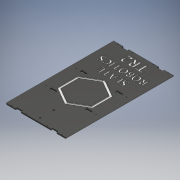
# Autodesk Inventor part: BA11
Saved by Autodesk Inventor 2017 (Build 210142000, 142)
## iProperties
Created: 2019-05-29
Part Number: BA11
Material: Wood (Cherry)
Document SubType Name: Modeling
Designer: Dell
Density: 0.63 g/cm^3
Appearance: Smooth - Black
Mass: 641.872 g
Surface Area: 3346.2 cm^2
Volume: 1018.84 cm^3
Author: Dell
Autodesk Inventor part; units mm, degrees
ref_plane "YZ Plane" through (0, 0, 0) normal (1, 0, 0) x (0, 1, 0)
ref_plane "XZ Plane" through (0, 0, 0) normal (0, 1, 0) x (-1, 0, 0)
ref_plane "XY Plane" through (0, 0, 0) normal (0, 0, 1) x (1, 0, 0)
sketch "Sketch1" plane through (0, 0, 0) normal (0, 0, 1) x (1, 0, 0)
  line L0 (0, 0) -> (303.5592, 0)
  line L1 (303.5592, 0) -> (303.5592, 539.75)
  line L2 (303.5592, 539.75) -> (0, 539.75)
  line L3 (0, 539.75) -> (0, 0)
  dimension "d0" = 539.75
  dimension "d1" = 303.5592
  constraints: 8 end point, 2 parallel, 1 horizontal, 1 perpendicular
  measures "d0" distance of L1.end L0.end
  measures "d1" distance of L1.end L2.end
extrude "Extrusion1" add sketch "Sketch1" along normal blind 6.35
sketch "Sketch2" plane through (0, 539.75, 0) normal (0, 1, 0) x (1, 0, 0)
  line L0 (0, -6.35) -> (303.5592, -6.35) projected
  line L1 (0, -6.35) -> (3.6662, 0)
  line L2 (0, 0) -> (303.5592, 0) projected
  line L3 (0, 0) -> (3.6662, 0)
  line L4 (0, 0) -> (0, -6.35)
  line L5 (303.5592, -6.35) -> (299.8931, 0)
  line L6 (303.5592, 0) -> (299.8931, 0)
  line L7 (303.5592, 0) -> (303.5592, -6.35) projected
  line L8 (303.5592, 0) -> (303.5592, -6.35)
  dimension "d4" = 30
  dimension "d5" = 30
  constraints: 12 end point, 2 collinear, 2 point on line, 1 perpendicular, 1 vertical
  measures "d4" angle of L4 L1
  measures "d5" angle of L5 L7
extrude "Extrusion2" cut sketch "Sketch2" against normal through all contours L4 L2 L1 | L5 L2 L7
sketch "Sketch3" plane through (0, 0, 6.35) normal (0, 0, 1) x (1, 0, 0)
  line L0 (50.1796, 532.13) -> (75.5796, 532.13)
  line L1 (75.5796, 532.13) -> (75.5796, 539.75)
  line L2 (75.5796, 539.75) -> (50.1796, 539.75)
  line L3 (50.1796, 539.75) -> (50.1796, 532.13)
  line L4 (303.5592, 539.75) -> (0, 539.75) projected
  line L5 (227.9796, 539.75) -> (253.3796, 539.75)
  line L6 (253.3796, 539.75) -> (253.3796, 532.13)
  line L7 (253.3796, 532.13) -> (227.9796, 532.13)
  line L8 (227.9796, 532.13) -> (227.9796, 539.75)
  line L9 (75.5796, 532.13) -> (227.9796, 532.13) construction
  line L10 (0, 0) -> (303.5592, 0) projected
  line L11 (50.1796, 0) -> (75.5796, 0)
  line L12 (75.5796, 0) -> (75.5796, 7.62)
  line L13 (75.5796, 7.62) -> (50.1796, 7.62)
  line L14 (50.1796, 7.62) -> (50.1796, 0)
  line L15 (253.3796, 0) -> (227.9796, 0)
  line L16 (227.9796, 0) -> (227.9796, 7.62)
  line L17 (227.9796, 7.62) -> (253.3796, 7.62)
  line L18 (253.3796, 7.62) -> (253.3796, 0)
  point P0 (151.7796, 532.13)
  point P1 (151.7796, 539.75)
  dimension "d8" = 7.62
  dimension "d9" = 25.4
  dimension "d10" = 25.4
  dimension "d11" = 152.4
  dimension "d14" = 7.62
  constraints: 34 end point, 8 parallel, 5 point on line, 5 vertical alignment, 4 horizontal, 4 perpendicular, 2 midpoint, 1 collinear, 1 horizontal alignment
  measures "d8" distance of L2.end L0.start
  measures "d9" distance of L0.start L0.end
  measures "d10" distance of L6.end L7.end
  measures "d11" distance of L0.end L7.end
  measures "d14" distance of L13.end L11.start
extrude "Extrusion3" cut sketch "Sketch3" against normal through all
sketch "Sketch4" plane through (0, 0, 6.35) normal (0, 0, 1) x (1, 0, 0)
  line L0 (50.1796, 330.2) -> (75.5796, 330.2)
  line L1 (75.5796, 330.2) -> (75.5796, 323.85)
  line L2 (75.5796, 323.85) -> (50.1796, 323.85)
  line L3 (50.1796, 323.85) -> (50.1796, 330.2)
  line L4 (227.9796, 330.2) -> (253.3796, 330.2)
  line L5 (253.3796, 330.2) -> (253.3796, 323.85)
  line L6 (253.3796, 323.85) -> (227.9796, 323.85)
  line L7 (227.9796, 323.85) -> (227.9796, 330.2)
  line L8 (75.5796, 532.13) -> (50.1796, 532.13) projected
  line L9 (253.3796, 532.13) -> (227.9796, 532.13) projected
  line L10 (227.9796, 539.75) -> (75.5796, 539.75) projected
  point P0 (0, 0)
  point P1 (62.8796, 330.2)
  point P2 (62.8796, 532.13)
  point P3 (240.6796, 330.2)
  point P4 (240.6796, 532.13)
  dimension "d15" = 25.4
  dimension "d16" = 6.35
  dimension "d17" = 25.4
  dimension "d18" = 6.35
  dimension "d19" = 209.55
  constraints: 16 end point, 4 midpoint, 4 parallel, 2 horizontal, 2 perpendicular, 2 vertical alignment, 1 horizontal alignment
  measures "d15" distance of L1.end L2.end
  measures "d16" distance of L0.end L1.end
  measures "d17" distance of L5.end L6.end
  measures "d18" distance of L4.end L5.end
  measures "d19" distance between parallel lines of L10 L0
extrude "Extrusion4" cut sketch "Sketch4" against normal through all
sketch "Sketch5" plane through (0, 0, 6.35) normal (0, 0, 1) x (1, 0, 0)
  line L0 (50.1796, 177.8) -> (75.5796, 177.8)
  line L1 (75.5796, 177.8) -> (75.5796, 171.45)
  line L2 (75.5796, 171.45) -> (50.1796, 171.45)
  line L3 (50.1796, 171.45) -> (50.1796, 177.8)
  line L4 (227.9796, 177.8) -> (253.3796, 177.8)
  line L5 (253.3796, 177.8) -> (253.3796, 171.45)
  line L6 (253.3796, 171.45) -> (227.9796, 171.45)
  line L7 (227.9796, 171.45) -> (227.9796, 177.8)
  line L8 (50.1796, 7.62) -> (75.5796, 7.62) projected
  line L9 (227.9796, 7.62) -> (253.3796, 7.62) projected
  line L10 (0, 0) -> (50.1796, 0) projected
  point P0 (62.8796, 171.45)
  point P1 (62.8796, 7.62)
  point P2 (240.6796, 7.62)
  point P3 (240.6796, 171.45)
  dimension "d22" = 25.4
  dimension "d23" = 6.35
  dimension "d24" = 25.4
  dimension "d25" = 6.35
  dimension "d27" = 177.8
  constraints: 16 end point, 4 midpoint, 4 parallel, 2 horizontal, 2 perpendicular, 2 vertical alignment, 1 horizontal alignment
  measures "d22" distance of L1.end L2.end
  measures "d23" distance of L0.end L1.end
  measures "d24" distance of L5.end L6.end
  measures "d25" distance of L4.end L5.end
  measures "d27" distance between parallel lines of L10 L0
extrude "Extrusion5" cut sketch "Sketch5" against normal through all
sketch "Sketch6" plane through (0, 0, 6.35) normal (0, 0, 1) x (1, 0, 0)
  line L0 (301.7796, 364.75) -> (1.7796, 364.75) construction
  line L1 (1.7796, 364.75) -> (1.7796, 514.75) construction
  line L2 (301.7796, 514.75) -> (301.7796, 364.75) construction
  line L3 (1.7796, 514.75) -> (301.7796, 514.75) construction
  line L4 (151.7796, 364.75) -> (151.7796, 439.75) construction
  line L5 (151.7796, 439.75) -> (1.7796, 439.75) construction
  line L6 (227.9796, 539.75) -> (75.5796, 539.75) projected
  line L7 (151.7796, 143.9637) -> (64.2796, 194.4819)
  line L8 (64.2796, 194.4819) -> (64.2796, 295.5181)
  line L9 (64.2796, 295.5181) -> (151.7796, 346.0363)
  line L10 (151.7796, 346.0363) -> (239.2796, 295.5181)
  line L11 (239.2796, 295.5181) -> (239.2796, 194.4819)
  line L12 (239.2796, 194.4819) -> (151.7796, 143.9637)
  line L13 (151.7796, 155.7416) -> (74.4796, 200.3708)
  line L14 (74.4796, 200.3708) -> (74.4796, 289.6292)
  line L15 (74.4796, 289.6292) -> (151.7796, 334.2584)
  line L16 (151.7796, 334.2584) -> (229.0796, 289.6292)
  line L17 (229.0796, 289.6292) -> (229.0796, 200.3708)
  line L18 (229.0796, 200.3708) -> (151.7796, 155.7416)
  line L19 (75.5796, 0) -> (227.9796, 0) projected
  line L20 (221.0068, 398.0391) -> (221.0068, 392.4691)
  spline S0 degree 2 poles (221.0068, 392.4691) (217.2023, 394.0605) (213.4476, 394.6822) (211.881, 394.6822) knots 0 0 0 1 2 2 2
  spline S1 degree 2 poles (211.881, 394.6822) (209.0463, 394.6822) (206.2364, 392.1458) (206.2364, 390.3555) knots 0 0 0 1 2 2 2
  spline S2 degree 2 poles (206.2364, 390.3555) (206.2364, 388.9878) (207.0072, 387.8937) knots 0 0 0 1 1 1
  spline S3 degree 2 poles (207.0072, 387.8937) (207.8029, 386.8245) (210.8615, 385.1087) knots 0 0 0 1 1 1
  line L21 (210.8615, 385.1087) -> (213.0497, 383.8903)
  spline S4 degree 2 poles (213.0497, 383.8903) (217.7494, 381.2793) (219.3906, 379.0663) knots 0 0 0 1 1 1
  spline S5 degree 2 poles (219.3906, 379.0663) (221.0814, 376.8532) (221.0814, 373.9438) knots 0 0 0 1 1 1
  spline S6 degree 2 poles (221.0814, 373.9438) (221.0814, 370.2637) (215.4617, 365.0418) (210.215, 365.0418) knots 0 0 0 1 2 2 2
  spline S7 degree 2 poles (210.215, 365.0418) (206.2861, 365.0418) (201.3626, 366.1607) knots 0 0 0 1 1 1
  line L22 (201.3626, 366.1607) -> (201.3626, 371.3578)
  spline S8 degree 2 poles (201.3626, 371.3578) (206.4104, 369.4928) (209.3695, 369.4928) knots 0 0 0 1 1 1
  spline S9 degree 2 poles (209.3695, 369.4928) (211.8313, 369.4928) (214.3925, 371.6313) (214.3925, 373.1233) knots 0 0 0 1 2 2 2
  spline S10 degree 2 poles (214.3925, 373.1233) (214.3925, 374.2671) (213.5968, 375.2369) knots 0 0 0 1 1 1
  spline S11 degree 2 poles (213.5968, 375.2369) (212.8508, 376.2315) (209.7922, 377.9473) knots 0 0 0 1 1 1
  line L23 (209.7922, 377.9473) -> (207.4548, 379.2403)
  spline S12 degree 2 poles (207.4548, 379.2403) (202.0589, 382.2491) (200.5918, 384.4622) knots 0 0 0 1 1 1
  spline S13 degree 2 poles (200.5918, 384.4622) (199.1247, 386.7002) (199.1247, 389.4852) knots 0 0 0 1 1 1
  spline S14 degree 2 poles (199.1247, 389.4852) (199.1247, 393.4886) (205.2169, 399.1332) (211.8561, 399.1332) knots 0 0 0 1 2 2 2
  spline S15 degree 2 poles (211.8561, 399.1332) (215.785, 399.1332) (221.0068, 398.0391) knots 0 0 0 1 1 1
  line L24 (193.5049, 398.3375) -> (193.5049, 365.8375)
  line L25 (193.5049, 365.8375) -> (186.7414, 365.8375)
  line L26 (186.7414, 365.8375) -> (186.7414, 393.7373)
  line L27 (186.7414, 393.7373) -> (172.2444, 393.7373)
  line L28 (172.2444, 393.7373) -> (172.2444, 398.3375)
  line L29 (172.2444, 398.3375) -> (193.5049, 398.3375)
  line L30 (170.9265, 398.3375) -> (158.3194, 365.8375)
  line L31 (158.3194, 365.8375) -> (151.531, 365.8375)
  line L32 (151.531, 365.8375) -> (138.8741, 398.3375)
  line L33 (138.8741, 398.3375) -> (145.8117, 398.3375)
  line L34 (145.8117, 398.3375) -> (149.1935, 389.6592)
  line L35 (149.1935, 389.6592) -> (162.6212, 389.6592)
  line L36 (162.6212, 389.6592) -> (166.003, 398.3375)
  line L37 (166.003, 398.3375) -> (170.9265, 398.3375)
  line L38 (160.9552, 385.3325) -> (150.8844, 385.3325)
  line L39 (150.8844, 385.3325) -> (155.9074, 372.3773)
  line L40 (155.9074, 372.3773) -> (160.9552, 385.3325)
  line L41 (126.1924, 398.3375) -> (126.1924, 370.3134)
  line L42 (126.1924, 370.3134) -> (137.8297, 370.3134)
  line L43 (137.8297, 370.3134) -> (137.8297, 365.8375)
  line L44 (137.8297, 365.8375) -> (107.7915, 365.8375)
  line L45 (107.7915, 365.8375) -> (107.7915, 370.3134)
  line L46 (107.7915, 370.3134) -> (119.4288, 370.3134)
  line L47 (119.4288, 370.3134) -> (119.4288, 398.3375)
  line L48 (119.4288, 398.3375) -> (126.1924, 398.3375)
  line L49 (103.2658, 398.3375) -> (103.2658, 365.8375)
  line L50 (103.2658, 365.8375) -> (82.4529, 365.8375)
  line L51 (82.4529, 365.8375) -> (82.4529, 370.3134)
  line L52 (82.4529, 370.3134) -> (96.5023, 370.3134)
  line L53 (96.5023, 370.3134) -> (96.5023, 379.3646)
  line L54 (96.5023, 379.3646) -> (84.8898, 379.3646)
  line L55 (84.8898, 379.3646) -> (84.8898, 383.8405)
  line L56 (84.8898, 383.8405) -> (96.5023, 383.8405)
  line L57 (96.5023, 383.8405) -> (96.5023, 393.7373)
  line L58 (96.5023, 393.7373) -> (81.4085, 393.7373)
  line L59 (81.4085, 393.7373) -> (81.4085, 398.3375)
  line L60 (81.4085, 398.3375) -> (103.2658, 398.3375)
  line L61 (266.201, 450.2809) -> (266.201, 417.7809)
  line L62 (266.201, 417.7809) -> (254.0415, 417.7809)
  spline S16 degree 2 poles (254.0415, 417.7809) (250.3116, 417.7809) (246.4076, 419.6459) (244.1448, 423.4504) (244.1448, 425.8376) knots 0 0 0 1 2 3 3 3
  spline S17 degree 2 poles (244.1448, 425.8376) (244.1448, 428.6972) (247.4271, 433.7699) (250.4359, 435.1126) knots 0 0 0 1 2 2 2
  line L63 (250.4359, 435.1126) -> (239.8181, 450.2809)
  line L64 (239.8181, 450.2809) -> (248.0487, 450.2809)
  line L65 (248.0487, 450.2809) -> (256.1302, 437.0024)
  line L66 (256.1302, 437.0024) -> (259.8353, 437.0024)
  line L67 (259.8353, 437.0024) -> (259.8353, 450.2809)
  line L68 (259.8353, 450.2809) -> (266.201, 450.2809)
  line L69 (259.8353, 432.5514) -> (258.2936, 432.5514)
  spline S18 degree 2 poles (258.2936, 432.5514) (254.1161, 432.5514) (250.9083, 428.8961) (250.9083, 426.5835) knots 0 0 0 1 2 2 2
  spline S19 degree 2 poles (250.9083, 426.5835) (250.9083, 424.5943) (253.4944, 422.232) (257.473, 422.232) knots 0 0 0 1 2 2 2
  line L70 (257.473, 422.232) -> (259.8353, 422.232)
  line L71 (259.8353, 422.232) -> (259.8353, 432.5514)
  spline S20 degree 2 poles (220.7209, 451.0767) (225.7936, 451.0767) (233.3031, 446.8743) (237.2071, 439.0166) (237.2071, 434.0185) knots 0 0 0 1 2 3 3 3
  spline S21 degree 2 poles (237.2071, 434.0185) (237.2071, 429.0702) (233.3031, 421.1627) (225.7438, 416.9852) (220.7209, 416.9852) knots 0 0 0 1 2 3 3 3
  spline S22 degree 2 poles (220.7209, 416.9852) (215.7228, 416.9852) (208.1635, 421.1627) (204.2595, 429.0702) (204.2595, 434.0185) knots 0 0 0 1 2 3 3 3
  spline S23 degree 2 poles (204.2595, 434.0185) (204.2595, 439.0166) (208.1635, 446.8743) (215.6482, 451.0767) (220.7209, 451.0767) knots 0 0 0 1 2 3 3 3
  spline S24 degree 2 poles (220.7209, 446.6256) (216.0212, 446.6256) (211.4458, 438.9669) (211.4458, 434.0185) knots 0 0 0 1 2 2 2
  spline S25 degree 2 poles (211.4458, 434.0185) (211.4458, 429.0453) (216.0461, 421.4363) (220.7209, 421.4363) knots 0 0 0 1 2 2 2
  spline S26 degree 2 poles (220.7209, 421.4363) (225.4206, 421.4363) (230.0208, 429.0453) (230.0208, 434.0185) knots 0 0 0 1 2 2 2
  spline S27 degree 2 poles (230.0208, 434.0185) (230.0208, 438.9669) (225.4454, 446.6256) (220.7209, 446.6256) knots 0 0 0 1 2 2 2
  line L72 (198.1922, 450.2809) -> (198.1922, 417.7809)
  line L73 (198.1922, 417.7809) -> (187.2262, 417.7809)
  spline S28 degree 2 poles (187.2262, 417.7809) (183.2477, 417.7809) (179.4432, 419.5713) (177.2798, 423.0526) (177.2798, 425.017) knots 0 0 0 1 2 3 3 3
  spline S29 degree 2 poles (177.2798, 425.017) (177.2798, 427.4539) (180.6616, 431.9298) (185.038, 433.2974) knots 0 0 0 1 2 2 2
  spline S30 degree 2 poles (185.038, 433.2974) (181.5568, 434.1677) (177.8766, 436.7041) (175.9619, 440.235) (175.9619, 442.2492) knots 0 0 0 1 2 3 3 3
  spline S31 degree 2 poles (175.9619, 442.2492) (175.9619, 444.4374) (178.1998, 448.2419) (182.1287, 450.2809) (186.2067, 450.2809) knots 0 0 0 1 2 3 3 3
  line L74 (186.2067, 450.2809) -> (198.1922, 450.2809)
  line L75 (191.7021, 445.6807) -> (190.4091, 445.6807)
  spline S32 degree 2 poles (190.4091, 445.6807) (186.8781, 445.6807) (184.3169, 444.7607) (183.0239, 442.6968) (183.0239, 441.4286) knots 0 0 0 1 2 3 3 3
  spline S33 degree 2 poles (183.0239, 441.4286) (183.0239, 439.0166) (187.276, 435.6597) (190.5334, 435.6597) knots 0 0 0 1 2 2 2
  line L76 (190.5334, 435.6597) -> (191.7021, 435.6597)
  line L77 (191.7021, 435.6597) -> (191.7021, 445.6807)
  line L78 (191.7021, 431.3081) -> (190.2599, 431.3081)
  spline S34 degree 2 poles (190.2599, 431.3081) (187.1765, 431.3081) (184.1428, 428.2496) (184.1428, 426.0614) knots 0 0 0 1 2 2 2
  spline S35 degree 2 poles (184.1428, 426.0614) (184.1428, 424.8927) (185.038, 423.1769) (187.3008, 422.232) (190.4837, 422.232) knots 0 0 0 1 2 3 3 3
  line L79 (190.4837, 422.232) -> (191.7021, 422.232)
  line L80 (191.7021, 422.232) -> (191.7021, 431.3081)
  spline S36 degree 2 poles (155.3976, 451.0767) (160.4703, 451.0767) (167.9799, 446.8743) (171.8839, 439.0166) (171.8839, 434.0185) knots 0 0 0 1 2 3 3 3
  spline S37 degree 2 poles (171.8839, 434.0185) (171.8839, 429.0702) (167.9799, 421.1627) (160.4206, 416.9852) (155.3976, 416.9852) knots 0 0 0 1 2 3 3 3
  spline S38 degree 2 poles (155.3976, 416.9852) (150.3995, 416.9852) (142.8402, 421.1627) (138.9363, 429.0702) (138.9363, 434.0185) knots 0 0 0 1 2 3 3 3
  spline S39 degree 2 poles (138.9363, 434.0185) (138.9363, 439.0166) (142.8402, 446.8743) (150.3249, 451.0767) (155.3976, 451.0767) knots 0 0 0 1 2 3 3 3
  spline S40 degree 2 poles (155.3976, 446.6256) (150.6979, 446.6256) (146.1226, 438.9669) (146.1226, 434.0185) knots 0 0 0 1 2 2 2
  spline S41 degree 2 poles (146.1226, 434.0185) (146.1226, 429.0453) (150.7228, 421.4363) (155.3976, 421.4363) knots 0 0 0 1 2 2 2
  spline S42 degree 2 poles (155.3976, 421.4363) (160.0973, 421.4363) (164.6976, 429.0453) (164.6976, 434.0185) knots 0 0 0 1 2 2 2
  spline S43 degree 2 poles (164.6976, 434.0185) (164.6976, 438.9669) (160.1222, 446.6256) (155.3976, 446.6256) knots 0 0 0 1 2 2 2
  line L81 (124.7875, 450.2809) -> (124.7875, 422.2568)
  line L82 (124.7875, 422.2568) -> (136.4248, 422.2568)
  line L83 (136.4248, 422.2568) -> (136.4248, 417.7809)
  line L84 (136.4248, 417.7809) -> (106.3865, 417.7809)
  line L85 (106.3865, 417.7809) -> (106.3865, 422.2568)
  line L86 (106.3865, 422.2568) -> (118.0239, 422.2568)
  line L87 (118.0239, 422.2568) -> (118.0239, 450.2809)
  line L88 (118.0239, 450.2809) -> (124.7875, 450.2809)
  line L89 (101.8609, 450.2809) -> (101.8609, 417.7809)
  line L90 (101.8609, 417.7809) -> (95.0973, 417.7809)
  line L91 (95.0973, 417.7809) -> (95.0973, 450.2809)
  line L92 (95.0973, 450.2809) -> (101.8609, 450.2809)
  spline S44 degree 2 poles (60.807, 448.9879) (62.9454, 449.9328) (66.1034, 450.6291) (70.1069, 451.0767) (72.0713, 451.0767) knots 0 0 0 1 2 3 3 3
  spline S45 degree 2 poles (72.0713, 451.0767) (80.6004, 451.0767) (88.9803, 441.4783) (88.9803, 434.0185) knots 0 0 0 1 2 2 2
  spline S46 degree 2 poles (88.9803, 434.0185) (88.9803, 426.5587) (80.6253, 416.9852) (71.6486, 416.9852) knots 0 0 0 1 2 2 2
  spline S47 degree 2 poles (71.6486, 416.9852) (66.3521, 416.9852) (61.1054, 418.2285) knots 0 0 0 1 1 1
  line L93 (61.1054, 418.2285) -> (61.1054, 423.525)
  spline S48 degree 2 poles (61.1054, 423.525) (63.6417, 422.6547) (66.8494, 421.8341) (69.709, 421.4363) (71.1513, 421.4363) knots 0 0 0 1 2 3 3 3
  spline S49 degree 2 poles (71.1513, 421.4363) (76.7461, 421.4363) (81.794, 428.6226) (81.794, 433.9439) knots 0 0 0 1 2 2 2
  spline S50 degree 2 poles (81.794, 433.9439) (81.794, 439.5139) (76.0748, 446.4018) (70.4053, 446.4018) knots 0 0 0 1 2 2 2
  spline S51 degree 2 poles (70.4053, 446.4018) (65.6807, 446.4018) (60.807, 444.0147) knots 0 0 0 1 1 1
  line L94 (60.807, 444.0147) -> (60.807, 448.9879)
  line L95 (56.7538, 449.9826) -> (56.7538, 444.4125)
  spline S52 degree 2 poles (56.7538, 444.4125) (52.9493, 446.004) (49.1945, 446.6256) (47.6279, 446.6256) knots 0 0 0 1 2 2 2
  spline S53 degree 2 poles (47.6279, 446.6256) (44.7932, 446.6256) (41.9833, 444.0893) (41.9833, 442.2989) knots 0 0 0 1 2 2 2
  spline S54 degree 2 poles (41.9833, 442.2989) (41.9833, 440.9313) (42.7542, 439.8372) knots 0 0 0 1 1 1
  spline S55 degree 2 poles (42.7542, 439.8372) (43.5499, 438.7679) (46.6084, 437.0522) knots 0 0 0 1 1 1
  line L96 (46.6084, 437.0522) -> (48.7966, 435.8337)
  spline S56 degree 2 poles (48.7966, 435.8337) (53.4963, 433.2228) (55.1375, 431.0097) knots 0 0 0 1 1 1
  spline S57 degree 2 poles (55.1375, 431.0097) (56.8284, 428.7966) (56.8284, 425.8873) knots 0 0 0 1 1 1
  spline S58 degree 2 poles (56.8284, 425.8873) (56.8284, 422.2071) (51.2086, 416.9852) (45.9619, 416.9852) knots 0 0 0 1 2 2 2
  spline S59 degree 2 poles (45.9619, 416.9852) (42.0331, 416.9852) (37.1096, 418.1042) knots 0 0 0 1 1 1
  line L97 (37.1096, 418.1042) -> (37.1096, 423.3012)
  spline S60 degree 2 poles (37.1096, 423.3012) (42.1574, 421.4363) (45.1165, 421.4363) knots 0 0 0 1 1 1
  spline S61 degree 2 poles (45.1165, 421.4363) (47.5782, 421.4363) (50.1394, 423.5748) (50.1394, 425.0667) knots 0 0 0 1 2 2 2
  spline S62 degree 2 poles (50.1394, 425.0667) (50.1394, 426.2106) (49.3437, 427.1803) knots 0 0 0 1 1 1
  spline S63 degree 2 poles (49.3437, 427.1803) (48.5977, 428.175) (45.5392, 429.8907) knots 0 0 0 1 1 1
  line L98 (45.5392, 429.8907) -> (43.2018, 431.1838)
  spline S64 degree 2 poles (43.2018, 431.1838) (37.8058, 434.1926) (36.3387, 436.4057) knots 0 0 0 1 1 1
  spline S65 degree 2 poles (36.3387, 436.4057) (34.8716, 438.6436) (34.8716, 441.4286) knots 0 0 0 1 1 1
  spline S66 degree 2 poles (34.8716, 441.4286) (34.8716, 445.4321) (40.9638, 451.0767) (47.6031, 451.0767) knots 0 0 0 1 2 2 2
  spline S67 degree 2 poles (47.6031, 451.0767) (51.5319, 451.0767) (56.7538, 449.9826) knots 0 0 0 1 1 1
  line L99 (195.2389, 514.4582) -> (195.2389, 477.8113)
  line L100 (195.2389, 477.8113) -> (210.4569, 477.8113)
  line L101 (210.4569, 477.8113) -> (210.4569, 471.9582)
  line L102 (210.4569, 471.9582) -> (171.1761, 471.9582)
  line L103 (171.1761, 471.9582) -> (171.1761, 477.8113)
  line L104 (171.1761, 477.8113) -> (186.3942, 477.8113)
  line L105 (186.3942, 477.8113) -> (186.3942, 514.4582)
  line L106 (186.3942, 514.4582) -> (195.2389, 514.4582)
  line L107 (165.258, 514.4582) -> (165.258, 471.9582)
  line L108 (165.258, 471.9582) -> (149.3571, 471.9582)
  spline S68 degree 2 poles (149.3571, 471.9582) (144.4795, 471.9582) (139.3743, 474.397) (136.4152, 479.3722) (136.4152, 482.4938) knots 0 0 0 1 2 3 3 3
  spline S69 degree 2 poles (136.4152, 482.4938) (136.4152, 486.2333) (140.7075, 492.8668) (144.6421, 494.6227) knots 0 0 0 1 2 2 2
  line L109 (144.6421, 494.6227) -> (130.7572, 514.4582)
  line L110 (130.7572, 514.4582) -> (141.5204, 514.4582)
  line L111 (141.5204, 514.4582) -> (152.0885, 497.094)
  line L112 (152.0885, 497.094) -> (156.9336, 497.094)
  line L113 (156.9336, 497.094) -> (156.9336, 514.4582)
  line L114 (156.9336, 514.4582) -> (165.258, 514.4582)
  line L115 (156.9336, 491.2735) -> (154.9175, 491.2735)
  spline S70 degree 2 poles (154.9175, 491.2735) (149.4546, 491.2735) (145.2599, 486.4934) (145.2599, 483.4693) knots 0 0 0 1 2 2 2
  spline S71 degree 2 poles (145.2599, 483.4693) (145.2599, 480.8679) (148.6417, 477.7788) (153.8445, 477.7788) knots 0 0 0 1 2 2 2
  line L116 (153.8445, 477.7788) -> (156.9336, 477.7788)
  line L117 (156.9336, 477.7788) -> (156.9336, 491.2735)
  line L118 (126.3999, 514.4582) -> (126.3999, 507.7272)
  spline S72 degree 2 poles (126.3999, 507.7272) (122.5629, 502.5569) (118.921, 499.4028) knots 0 0 0 1 1 1
  line L119 (118.921, 499.4028) -> (115.4416, 496.3461)
  spline S73 degree 2 poles (115.4416, 496.3461) (111.7021, 493.0294) (106.8246, 486.591) (106.8246, 483.0791) knots 0 0 0 1 2 2 2
  spline S74 degree 2 poles (106.8246, 483.0791) (106.8246, 479.8924) (110.9542, 476.4131) (114.4336, 476.4131) knots 0 0 0 1 2 2 2
  spline S75 degree 2 poles (114.4336, 476.4131) (119.1161, 476.4131) (125.2943, 479.5673) knots 0 0 0 1 1 1
  line L120 (125.2943, 479.5673) -> (125.2943, 473.3239)
  spline S76 degree 2 poles (125.2943, 473.3239) (118.7909, 470.9177) (112.7427, 470.9177) knots 0 0 0 1 1 1
  spline S77 degree 2 poles (112.7427, 470.9177) (106.0441, 470.9177) (97.8173, 477.3236) (97.8173, 482.6889) knots 0 0 0 1 2 2 2
  spline S78 degree 2 poles (97.8173, 482.6889) (97.8173, 486.0707) (101.2966, 492.0539) (106.7595, 496.4762) knots 0 0 0 1 2 2 2
  line L121 (106.7595, 496.4762) -> (109.6536, 498.7849)
  spline S79 degree 2 poles (109.6536, 498.7849) (111.5396, 500.3132) (116.0594, 505.0608) (116.7748, 507.7272) knots 0 0 0 1 2 2 2
  line L122 (116.7748, 507.7272) -> (97.9799, 507.7272)
  line L123 (97.9799, 507.7272) -> (97.9799, 514.4582)
  line L124 (97.9799, 514.4582) -> (126.3999, 514.4582)
  point P0 (0, 0)
  point P1 (151.7796, 514.75)
  point P2 (151.7796, 539.75)
  point P3 (151.7796, 245)
  dimension "d32" = 300
  dimension "d34" = 175
  dimension "d35" = 10.2
  dimension "d38" = 245
  dimension "d39" = 100
  dimension "d40" = 150
  constraints: 28 end point, 4 midpoint, 2 horizontal, 2 vertical, 2 vertical alignment, 20 other
  measures "d32" distance of L2.end L0.end
  measures "d34" distance between parallel lines of L11 L8
  measures "d35" distance between parallel lines of L12 L18
  measures "d38" distance from line of point (151.78, 245) L19
  measures "d39" distance from line of L6 L4.end
  measures "d40" distance of L2.start L2.end
extrude "Extrusion6" cut sketch "Sketch6" against normal blind 3.175
sketch "Sketch7" plane through (0, 0, 6.35) normal (0, 0, 1) x (1, 0, 0)
  line L0 (26.2013, 535.94) -> (99.558, 535.94) construction
  line L1 (75.5796, 532.13) -> (50.1796, 532.13) construction
  line L2 (50.1796, 532.13) -> (50.1796, 539.75) construction
  line L3 (204.0013, 535.94) -> (277.358, 535.94) construction
  line L4 (253.3796, 532.13) -> (227.9796, 532.13) construction
  circle A0 centre (26.2013, 535.94) radius 2.25
  circle A1 centre (99.558, 535.94) radius 2.25
  circle A2 centre (204.0013, 535.94) radius 2.25
  circle A3 centre (277.358, 535.94) radius 2.25
  circle A4 centre (26.2013, 327.025) radius 2.25
  circle A5 centre (99.558, 327.025) radius 2.25
  circle A6 centre (204.0013, 327.025) radius 2.25
  circle A7 centre (277.358, 327.025) radius 2.25
  circle A8 centre (277.358, 174.625) radius 2.25
  circle A9 centre (26.2013, 174.625) radius 2.25
  circle A10 centre (151.7796, 174.625) radius 2.25
  circle A11 centre (26.2013, 3.81) radius 2.25
  circle A12 centre (99.558, 3.81) radius 2.25
  circle A13 centre (204.0013, 3.81) radius 2.25
  circle A14 centre (277.358, 3.81) radius 2.25
  line L5 (227.9796, 539.75) -> (75.5796, 539.75) projected
  line L6 (50.1796, 323.85) -> (50.1796, 330.2) projected
  line L7 (50.1796, 171.45) -> (50.1796, 177.8) projected
  line L8 (50.1796, 0) -> (50.1796, 7.62) projected
  point P0 (0, 0)
  point P1 (62.8796, 535.94)
  point P2 (62.8796, 532.13)
  point P3 (50.1796, 535.94)
  point P4 (240.6796, 535.94)
  point P5 (240.6796, 532.13)
  point P6 (151.7796, 539.75)
  point P7 (50.1796, 327.025)
  point P8 (50.1796, 174.625)
  point P9 (50.1796, 3.81)
  dimension "d41" = 73.3567
  dimension "d42" = 73.3567
  dimension "d43" = 4.5
  dimension "d44" = 4.5
  dimension "d45" = 4.5
  dimension "d46" = 4.5
  dimension "d47" = 4.5
  dimension "d48" = 4.5
  dimension "d49" = 4.5
  dimension "d50" = 4.5
  dimension "d51" = 4.5
  dimension "d52" = 4.5
  dimension "d53" = 4.5
  dimension "d54" = 4.5
  dimension "d55" = 4.5
  dimension "d56" = 4.5
  dimension "d57" = 4.5
  constraints: 15 centre point, 13 horizontal alignment, 13 vertical alignment, 9 midpoint, 4 coincident, 4 end point, 2 horizontal
  measures "d41" distance of L0.start L0.end
  measures "d42" distance of L3.start L3.end
  measures "d43" diameter of A0
  measures "d44" diameter of A1
  measures "d45" diameter of A2
  measures "d46" diameter of A3
  measures "d47" diameter of A4
  measures "d48" diameter of A5
  measures "d49" diameter of A6
  measures "d50" diameter of A7
  measures "d51" diameter of A8
  measures "d52" diameter of A9
  measures "d53" diameter of A10
  measures "d54" diameter of A11
  measures "d55" diameter of A12
  measures "d56" diameter of A13
  measures "d57" diameter of A14
extrude "Extrusion7" cut sketch "Sketch7" against normal through all contours A0 | A1 | A2 | A3 | A4 | A7 | A8 | A9 | A11 | A12 | A13 | A14
sketch "Sketch8" plane through (0, 0, 6.35) normal (0, 0, 1) x (1, 0, 0)
  circle A0 centre (151.7796, 20) radius 4
  circle A1 centre (151.7796, 87.71) radius 4
  line L0 (75.5796, 0) -> (227.9796, 0) projected
  point P0 (0, 0)
  point P1 (151.7796, 0)
  point P2 (151.7796, 0)
  dimension "d60" = 8
  dimension "d61" = 8
  dimension "d63" = 20
  dimension "d64" = 67.71
  constraints: 2 centre point, 2 midpoint, 2 vertical alignment
  measures "d60" diameter of A0
  measures "d61" diameter of A1
  measures "d63" distance from line of L0 A0.centre
  measures "d64" distance of A1.centre A0.centre
extrude "Extrusion8" cut sketch "Sketch8" against normal through all
sketch "Sketch9" plane through (0, 0, 6.35) normal (0, 0, 1) x (1, 0, 0)
  line L0 (50.1796, 539.75) -> (3.6662, 539.75) projected
  line L1 (48.9096, 539.75) -> (76.8496, 539.75)
  line L2 (76.8496, 539.75) -> (76.8496, 532.13)
  line L3 (76.8496, 532.13) -> (48.9096, 532.13)
  line L4 (48.9096, 532.13) -> (48.9096, 539.75)
  line L5 (227.9796, 539.75) -> (75.5796, 539.75) projected
  line L6 (226.7096, 539.75) -> (254.6496, 539.75)
  line L7 (254.6496, 539.75) -> (254.6496, 532.13)
  line L8 (254.6496, 532.13) -> (226.7096, 532.13)
  line L9 (226.7096, 532.13) -> (226.7096, 539.75)
  line L10 (48.9096, 331.47) -> (76.8496, 331.47)
  line L11 (76.8496, 331.47) -> (76.8496, 322.58)
  line L12 (76.8496, 322.58) -> (48.9096, 322.58)
  line L13 (48.9096, 322.58) -> (48.9096, 331.47)
  line L14 (48.9096, 179.07) -> (76.8496, 179.07)
  line L15 (76.8496, 179.07) -> (76.8496, 170.18)
  line L16 (76.8496, 170.18) -> (48.9096, 170.18)
  line L17 (48.9096, 170.18) -> (48.9096, 179.07)
  line L18 (254.6496, 170.18) -> (226.7096, 170.18)
  line L19 (226.7096, 170.18) -> (226.7096, 179.07)
  line L20 (226.7096, 179.07) -> (254.6496, 179.07)
  line L21 (254.6496, 179.07) -> (254.6496, 170.18)
  line L22 (254.6496, 322.58) -> (226.7096, 322.58)
  line L23 (226.7096, 322.58) -> (226.7096, 331.47)
  line L24 (226.7096, 331.47) -> (254.6496, 331.47)
  line L25 (254.6496, 331.47) -> (254.6496, 322.58)
  line L26 (3.6662, 0) -> (50.1796, 0) projected
  line L27 (48.9096, 0) -> (76.8496, 0)
  line L28 (76.8496, 0) -> (76.8496, 7.62)
  line L29 (76.8496, 7.62) -> (48.9096, 7.62)
  line L30 (48.9096, 7.62) -> (48.9096, 0)
  line L31 (75.5796, 0) -> (227.9796, 0) projected
  line L32 (226.7096, 0) -> (254.6496, 0)
  line L33 (254.6496, 0) -> (254.6496, 7.62)
  line L34 (254.6496, 7.62) -> (226.7096, 7.62)
  line L35 (226.7096, 7.62) -> (226.7096, 0)
  line L36 (50.1796, 7.62) -> (75.5796, 7.62) projected
  line L37 (227.9796, 7.62) -> (253.3796, 7.62) projected
  line L38 (253.3796, 532.13) -> (227.9796, 532.13) projected
  line L39 (75.5796, 532.13) -> (50.1796, 532.13) projected
  line L40 (50.1796, 532.13) -> (50.1796, 539.75) projected
  line L41 (227.9796, 532.13) -> (227.9796, 539.75) projected
  line L42 (227.9796, 0) -> (227.9796, 7.62) projected
  line L43 (50.1796, 0) -> (50.1796, 7.62) projected
  line L44 (50.1796, 177.8) -> (75.5796, 177.8) projected
  line L45 (227.9796, 177.8) -> (253.3796, 177.8) projected
  line L46 (50.1796, 330.2) -> (75.5796, 330.2) projected
  line L47 (227.9796, 323.85) -> (227.9796, 330.2) projected
  line L48 (75.5796, 330.2) -> (75.5796, 323.85) projected
  line L49 (227.9796, 171.45) -> (227.9796, 177.8) projected
  line L50 (75.5796, 177.8) -> (75.5796, 171.45) projected
  line L51 (227.9796, 330.2) -> (253.3796, 330.2) projected
  point P0 (0, 0)
  point P1 (62.8796, 7.62)
  point P2 (62.8796, 7.62)
  point P3 (240.6796, 7.62)
  point P4 (240.6796, 532.13)
  point P5 (62.8796, 532.13)
  point P6 (75.5796, 327.025)
  point P7 (76.8496, 327.025)
  point P8 (227.9796, 174.625)
  point P9 (226.7096, 174.625)
  point P10 (75.5796, 174.625)
  point P11 (76.8496, 174.625)
  point P12 (62.8796, 330.2)
  point P13 (62.8796, 331.47)
  point P14 (240.6796, 330.2)
  point P15 (240.6796, 331.47)
  point P16 (62.8796, 177.8)
  point P17 (62.8796, 179.07)
  point P18 (62.8796, 177.8)
  dimension "d68" = 1.27
  dimension "d69" = 1.27
  dimension "d70" = 1.27
  dimension "d71" = 1.27
  dimension "d72" = 1.27
  dimension "d73" = 1.27
  dimension "d74" = 1.27
  dimension "d75" = 1.27
  constraints: 64 end point, 23 midpoint, 16 parallel, 11 point on line, 8 horizontal, 8 perpendicular, 3 horizontal alignment, 3 vertical alignment
  measures "d68" distance between parallel lines of L4 L40
  measures "d69" distance between parallel lines of L41 L9
  measures "d70" distance between parallel lines of L42 L35
  measures "d71" distance between parallel lines of L30 L43
  measures "d72" distance between parallel lines of L14 L44
  measures "d73" distance between parallel lines of L20 L45
  measures "d74" distance between parallel lines of L10 L46
  measures "d75" distance between parallel lines of L23 L47
extrude "Extrusion9" cut sketch "Sketch9" against normal through all
sketch "Sketch10" plane through (0, 0, 6.35) normal (0, 0, 1) x (1, 0, 0)
  line L0 (76.8496, 7.62) -> (76.8496, 0) construction
  line L1 (76.8496, 0) -> (226.7096, 0) construction
  line L2 (226.7096, 0) -> (226.7096, 7.62) construction
  line L3 (226.7096, 7.62) -> (254.6496, 7.62) construction
  line L4 (254.6496, 7.62) -> (254.6496, 0) construction
  line L5 (254.6496, 0) -> (303.5592, 0) construction
  line L6 (303.5592, 0) -> (303.5592, 539.75) construction
  line L7 (303.5592, 539.75) -> (254.6496, 539.75) construction
  line L8 (254.6496, 539.75) -> (254.6496, 532.13) construction
  line L9 (254.6496, 532.13) -> (226.7096, 532.13) construction
  line L10 (226.7096, 532.13) -> (226.7096, 539.75) construction
  line L11 (226.7096, 539.75) -> (76.8496, 539.75) construction
  line L12 (76.8496, 539.75) -> (76.8496, 532.13) construction
  line L13 (76.8496, 532.13) -> (48.9096, 532.13) construction
  line L14 (48.9096, 532.13) -> (48.9096, 539.75) construction
  line L15 (48.9096, 539.75) -> (0, 539.75) construction
  line L16 (0, 539.75) -> (0, 0) construction
  line L17 (0, 0) -> (48.9096, 0) construction
  line L18 (48.9096, 0) -> (48.9096, 7.62) construction
  line L19 (48.9096, 7.62) -> (76.8496, 7.62) construction
  line L20 (254.6496, 179.07) -> (254.6496, 170.18) construction
  line L21 (254.6496, 170.18) -> (226.7096, 170.18) construction
  line L22 (226.7096, 170.18) -> (226.7096, 179.07) construction
  line L23 (226.7096, 179.07) -> (254.6496, 179.07) construction
  line L24 (48.9096, 322.58) -> (48.9096, 331.47) construction
  line L25 (48.9096, 331.47) -> (76.8496, 331.47) construction
  line L26 (76.8496, 331.47) -> (76.8496, 322.58) construction
  line L27 (76.8496, 322.58) -> (48.9096, 322.58) construction
  line L28 (48.9096, 170.18) -> (48.9096, 179.07) construction
  line L29 (48.9096, 179.07) -> (76.8496, 179.07) construction
  line L30 (76.8496, 179.07) -> (76.8496, 170.18) construction
  line L31 (76.8496, 170.18) -> (48.9096, 170.18) construction
  line L32 (254.6496, 331.47) -> (254.6496, 322.58) construction
  line L33 (254.6496, 322.58) -> (226.7096, 322.58) construction
  line L34 (226.7096, 322.58) -> (226.7096, 331.47) construction
  line L35 (226.7096, 331.47) -> (254.6496, 331.47) construction
  circle A0 centre (151.7796, 20) radius 4 construction
  circle A1 centre (151.7796, 87.71) radius 4 construction
  circle A2 centre (204.0013, 3.81) radius 2.25 construction
  circle A3 centre (26.2013, 3.81) radius 2.25 construction
  circle A4 centre (277.358, 174.625) radius 2.25 construction
  circle A5 centre (26.2013, 327.025) radius 2.25 construction
  circle A6 centre (204.0013, 535.94) radius 2.25 construction
  circle A7 centre (26.2013, 535.94) radius 2.25 construction
  circle A8 centre (99.558, 535.94) radius 2.25 construction
  circle A9 centre (277.358, 535.94) radius 2.25 construction
  circle A10 centre (277.358, 327.025) radius 2.25 construction
  circle A11 centre (26.2013, 174.625) radius 2.25 construction
  circle A12 centre (99.558, 3.81) radius 2.25 construction
  circle A13 centre (277.358, 3.81) radius 2.25 construction
  line L36 (186.3942, 514.4582) -> (195.2389, 514.4582) construction
  line L37 (195.2389, 514.4582) -> (195.2389, 477.8113) construction
  line L38 (195.2389, 477.8113) -> (210.4569, 477.8113) construction
  line L39 (210.4569, 477.8113) -> (210.4569, 471.9582) construction
  line L40 (210.4569, 471.9582) -> (171.1761, 471.9582) construction
  line L41 (171.1761, 471.9582) -> (171.1761, 477.8113) construction
  line L42 (171.1761, 477.8113) -> (186.3942, 477.8113) construction
  line L43 (186.3942, 477.8113) -> (186.3942, 514.4582) construction
  line L44 (60.807, 444.0147) -> (60.807, 448.9879) construction
  line L45 (61.1054, 418.2285) -> (61.1054, 423.525) construction
  line L46 (118.0239, 450.2809) -> (124.7875, 450.2809) construction
  line L47 (124.7875, 450.2809) -> (124.7875, 422.2568) construction
  line L48 (124.7875, 422.2568) -> (136.4248, 422.2568) construction
  line L49 (136.4248, 422.2568) -> (136.4248, 417.7809) construction
  line L50 (136.4248, 417.7809) -> (106.3865, 417.7809) construction
  line L51 (106.3865, 417.7809) -> (106.3865, 422.2568) construction
  line L52 (106.3865, 422.2568) -> (118.0239, 422.2568) construction
  line L53 (118.0239, 422.2568) -> (118.0239, 450.2809) construction
  line L54 (81.4085, 398.3375) -> (103.2658, 398.3375) construction
  line L55 (103.2658, 398.3375) -> (103.2658, 365.8375) construction
  line L56 (103.2658, 365.8375) -> (82.4529, 365.8375) construction
  line L57 (82.4529, 365.8375) -> (82.4529, 370.3134) construction
  line L58 (82.4529, 370.3134) -> (96.5023, 370.3134) construction
  line L59 (96.5023, 370.3134) -> (96.5023, 379.3646) construction
  line L60 (96.5023, 379.3646) -> (84.8898, 379.3646) construction
  line L61 (84.8898, 379.3646) -> (84.8898, 383.8405) construction
  line L62 (84.8898, 383.8405) -> (96.5023, 383.8405) construction
  line L63 (96.5023, 383.8405) -> (96.5023, 393.7373) construction
  line L64 (96.5023, 393.7373) -> (81.4085, 393.7373) construction
  line L65 (81.4085, 393.7373) -> (81.4085, 398.3375) construction
  line L66 (172.2444, 398.3375) -> (193.5049, 398.3375) construction
  line L67 (193.5049, 398.3375) -> (193.5049, 365.8375) construction
  line L68 (193.5049, 365.8375) -> (186.7414, 365.8375) construction
  line L69 (186.7414, 365.8375) -> (186.7414, 393.7373) construction
  line L70 (186.7414, 393.7373) -> (172.2444, 393.7373) construction
  line L71 (172.2444, 393.7373) -> (172.2444, 398.3375) construction
  line L72 (239.2796, 194.4819) -> (151.7796, 143.9637) construction
  line L73 (151.7796, 143.9637) -> (64.2796, 194.4819) construction
  line L74 (64.2796, 194.4819) -> (64.2796, 295.5181) construction
  line L75 (64.2796, 295.5181) -> (151.7796, 346.0363) construction
  line L76 (151.7796, 346.0363) -> (239.2796, 295.5181) construction
  line L77 (239.2796, 295.5181) -> (239.2796, 194.4819) construction
  line L78 (221.0068, 398.0391) -> (221.0068, 392.4691) construction
  line L79 (210.8615, 385.1087) -> (213.0497, 383.8903) construction
  line L80 (201.3626, 366.1607) -> (201.3626, 371.3578) construction
  line L81 (209.7922, 377.9473) -> (207.4548, 379.2403) construction
  line L82 (166.003, 398.3375) -> (170.9265, 398.3375) construction
  line L83 (170.9265, 398.3375) -> (158.3194, 365.8375) construction
  line L84 (158.3194, 365.8375) -> (151.531, 365.8375) construction
  line L85 (151.531, 365.8375) -> (138.8741, 398.3375) construction
  line L86 (138.8741, 398.3375) -> (145.8117, 398.3375) construction
  line L87 (145.8117, 398.3375) -> (149.1935, 389.6592) construction
  line L88 (149.1935, 389.6592) -> (162.6212, 389.6592) construction
  line L89 (162.6212, 389.6592) -> (166.003, 398.3375) construction
  line L90 (119.4288, 398.3375) -> (126.1924, 398.3375) construction
  line L91 (126.1924, 398.3375) -> (126.1924, 370.3134) construction
  line L92 (126.1924, 370.3134) -> (137.8297, 370.3134) construction
  line L93 (137.8297, 370.3134) -> (137.8297, 365.8375) construction
  line L94 (137.8297, 365.8375) -> (107.7915, 365.8375) construction
  line L95 (107.7915, 365.8375) -> (107.7915, 370.3134) construction
  line L96 (107.7915, 370.3134) -> (119.4288, 370.3134) construction
  line L97 (119.4288, 370.3134) -> (119.4288, 398.3375) construction
  line L98 (259.8353, 450.2809) -> (266.201, 450.2809) construction
  line L99 (266.201, 450.2809) -> (266.201, 417.7809) construction
  line L100 (266.201, 417.7809) -> (254.0415, 417.7809) construction
  line L101 (250.4359, 435.1126) -> (239.8181, 450.2809) construction
  line L102 (239.8181, 450.2809) -> (248.0487, 450.2809) construction
  line L103 (248.0487, 450.2809) -> (256.1302, 437.0024) construction
  line L104 (256.1302, 437.0024) -> (259.8353, 437.0024) construction
  line L105 (259.8353, 437.0024) -> (259.8353, 450.2809) construction
  line L106 (186.2067, 450.2809) -> (198.1922, 450.2809) construction
  line L107 (198.1922, 450.2809) -> (198.1922, 417.7809) construction
  line L108 (198.1922, 417.7809) -> (187.2262, 417.7809) construction
  line L109 (95.0973, 450.2809) -> (101.8609, 450.2809) construction
  line L110 (101.8609, 450.2809) -> (101.8609, 417.7809) construction
  line L111 (101.8609, 417.7809) -> (95.0973, 417.7809) construction
  line L112 (95.0973, 417.7809) -> (95.0973, 450.2809) construction
  line L113 (56.7538, 449.9826) -> (56.7538, 444.4125) construction
  line L114 (46.6084, 437.0522) -> (48.7966, 435.8337) construction
  line L115 (37.1096, 418.1042) -> (37.1096, 423.3012) construction
  line L116 (45.5392, 429.8907) -> (43.2018, 431.1838) construction
  line L117 (156.9336, 514.4582) -> (165.258, 514.4582) construction
  line L118 (165.258, 514.4582) -> (165.258, 471.9582) construction
  line L119 (165.258, 471.9582) -> (149.3571, 471.9582) construction
  line L120 (144.6421, 494.6227) -> (130.7572, 514.4582) construction
  line L121 (130.7572, 514.4582) -> (141.5204, 514.4582) construction
  line L122 (141.5204, 514.4582) -> (152.0885, 497.094) construction
  line L123 (152.0885, 497.094) -> (156.9336, 497.094) construction
  line L124 (156.9336, 497.094) -> (156.9336, 514.4582) construction
  line L125 (126.3999, 514.4582) -> (126.3999, 507.7272) construction
  line L126 (118.921, 499.4028) -> (115.4416, 496.3461) construction
  line L127 (119.1811, 474.5466) -> (118.2356, 469.8191) construction
  line L128 (97.9799, 507.7272) -> (97.9799, 514.4582) construction
  line L129 (305.8043, 541.9951) -> (305.8043, -2.2451) construction
  line L130 (305.8043, -2.2451) -> (252.4045, -2.2451) construction
  line L131 (252.4045, -2.2451) -> (252.4045, 5.3749) construction
  line L132 (252.4045, 5.3749) -> (228.9547, 5.3749) construction
  line L133 (228.9547, 5.3749) -> (228.9547, -2.2451) construction
  line L134 (228.9547, -2.2451) -> (74.6045, -2.2451) construction
  line L135 (74.6045, -2.2451) -> (74.6045, 5.3749) construction
  line L136 (74.6045, 5.3749) -> (51.1547, 5.3749) construction
  line L137 (51.1547, 5.3749) -> (51.1547, -2.2451) construction
  line L138 (51.1547, -2.2451) -> (-2.2451, -2.2451) construction
  line L139 (-2.2451, -2.2451) -> (-2.2451, 541.9951) construction
  line L140 (-2.2451, 541.9951) -> (51.1547, 541.9951) construction
  line L141 (51.1547, 541.9951) -> (51.1547, 534.3751) construction
  line L142 (51.1547, 534.3751) -> (74.6045, 534.3751) construction
  line L143 (74.6045, 534.3751) -> (74.6045, 541.9951) construction
  line L144 (74.6045, 541.9951) -> (228.9547, 541.9951) construction
  line L145 (228.9547, 541.9951) -> (228.9547, 534.3751) construction
  line L146 (228.9547, 534.3751) -> (252.4045, 534.3751) construction
  line L147 (252.4045, 534.3751) -> (252.4045, 541.9951) construction
  line L148 (252.4045, 541.9951) -> (305.8043, 541.9951) construction
  line L149 (252.4045, 329.2249) -> (252.4045, 324.8251) construction
  line L150 (252.4045, 324.8251) -> (228.9547, 324.8251) construction
  line L151 (228.9547, 324.8251) -> (228.9547, 329.2249) construction
  line L152 (228.9547, 329.2249) -> (252.4045, 329.2249) construction
  line L153 (252.4045, 176.8249) -> (252.4045, 172.4251) construction
  line L154 (252.4045, 172.4251) -> (228.9547, 172.4251) construction
  line L155 (228.9547, 172.4251) -> (228.9547, 176.8249) construction
  line L156 (228.9547, 176.8249) -> (252.4045, 176.8249) construction
  line L157 (74.6045, 176.8249) -> (51.1547, 176.8249) construction
  line L158 (51.1547, 176.8249) -> (51.1547, 172.4251) construction
  line L159 (51.1547, 172.4251) -> (74.6045, 172.4251) construction
  line L160 (74.6045, 172.4251) -> (74.6045, 176.8249) construction
  line L161 (74.6045, 329.2249) -> (51.1547, 329.2249) construction
  line L162 (51.1547, 329.2249) -> (51.1547, 324.8251) construction
  line L163 (51.1547, 324.8251) -> (74.6045, 324.8251) construction
  line L164 (74.6045, 324.8251) -> (74.6045, 329.2249) construction
  line L165 (254.6496, 532.13) -> (226.7096, 532.13) projected
  circle A14 centre (228.9547, 534.3751) radius 3.175
  circle A15 centre (252.4045, 534.3751) radius 3.175
  circle A16 centre (74.6045, 534.3751) radius 3.175
  circle A17 centre (51.1547, 534.3751) radius 3.175
  line L166 (226.7096, 7.62) -> (226.7096, 0) projected
  circle A18 centre (228.9547, 5.3749) radius 3.175
  circle A19 centre (252.4045, 5.3749) radius 3.175
  circle A20 centre (51.1547, 5.3749) radius 3.175
  circle A21 centre (74.6045, 5.3749) radius 3.175
  line L167 (48.9096, 179.07) -> (76.8496, 179.07) projected
  circle A22 centre (51.1547, 176.8249) radius 3.175
  circle A23 centre (51.1547, 172.4251) radius 3.175
  circle A24 centre (74.6045, 172.4251) radius 3.175
  circle A25 centre (74.6045, 176.8249) radius 3.175
  circle A26 centre (51.1547, 329.2249) radius 3.175
  circle A27 centre (51.1547, 324.8251) radius 3.175
  line L168 (76.8496, 322.58) -> (48.9096, 322.58) projected
  circle A28 centre (74.6045, 324.8251) radius 3.175
  circle A29 centre (74.6045, 329.2249) radius 3.175
  circle A30 centre (228.9547, 329.2249) radius 3.175
  circle A31 centre (228.9547, 324.8251) radius 3.175
  circle A32 centre (252.4045, 329.2249) radius 3.175
  circle A33 centre (252.4045, 324.8251) radius 3.175
  circle A34 centre (228.9547, 176.8249) radius 3.175
  circle A35 centre (228.9547, 172.4251) radius 3.175
  circle A36 centre (252.4045, 172.4251) radius 3.175
  line L169 (254.6496, 179.07) -> (254.6496, 170.18) projected
  circle A37 centre (252.4045, 176.8249) radius 3.175
  dimension "d78" = 6.35
  dimension "d79" = 6.35
  dimension "d80" = 6.35
  dimension "d81" = 6.35
  dimension "d82" = 6.35
  constraints: 72 end point, 23 coincident, 2 horizontal alignment, 1 vertical alignment, 167 other
extrude "Extrusion10" cut sketch "Sketch10" against normal through all
sketch "Sketch11" plane through (76.8496, 0, 0) normal (0, -1, 0) x (1, 0, 0)
  line L0 (-76.8496, 6.35) -> (-73.1834, 0) projected
  line L1 (223.0434, 0) -> (226.7096, 6.35) projected
  line L2 (-76.8496, 6.35) -> (-27.94, 6.35) projected
  line L3 (-76.8496, 6.35) -> (-76.1164, 6.35)
  line L4 (-76.1164, 6.35) -> (-72.4502, 0)
  line L5 (-73.1834, 0) -> (-27.94, 0) projected
  line L6 (-72.4502, 0) -> (-73.1834, 0)
  line L7 (226.7096, 6.35) -> (225.9764, 6.35)
  line L8 (177.8, 6.35) -> (226.7096, 6.35) projected
  line L9 (225.9764, 6.35) -> (222.3102, 0)
  line L10 (177.8, 0) -> (223.0434, 0) projected
  line L11 (222.3102, 0) -> (223.0434, 0)
  point P0 (-76.8496, 0)
  dimension "d85" = 0.635
  dimension "d86" = 0.635
  constraints: 12 end point, 4 point on line, 2 collinear, 1 parallel
  measures "d85" distance between parallel lines of L1 L9
  measures "d86" distance between parallel lines of L0 L4
extrude "Extrusion11" cut sketch "Sketch11" against normal through all
equation "\"d2\" = Panel_Thickness"
equation "\"d8\" = Panel_Thickness + Fit_Tolerance"
equation "\"d14\" = Panel_Thickness + Fit_Tolerance"
equation "\"d16\" = Panel_Thickness"
equation "\"d18\" = Panel_Thickness"
equation "\"d23\" = Panel_Thickness"
equation "\"d25\" = Panel_Thickness"
equation "\"d68\" = Fit_Tolerance"
equation "\"d69\" = Fit_Tolerance"
equation "\"d70\" = Fit_Tolerance"
equation "\"d71\" = Fit_Tolerance"
equation "\"d72\" = Fit_Tolerance"
equation "\"d73\" = Fit_Tolerance"
equation "\"d74\" = Fit_Tolerance"
equation "\"d75\" = Fit_Tolerance"
equation "\"d78\" = Tool_Dia"
equation "\"d79\" = Tool_Dia"
equation "\"d80\" = Tool_Dia"
equation "\"d81\" = Tool_Dia"
equation "\"d82\" = Tool_Dia"
equation "\"d85\" = 0.5 * Fit_Tolerance"
equation "\"d86\" = 0.5 * Fit_Tolerance"
equation "\"Panel_Thickness\" = 6.35"
equation "\"Fit_Tolerance\" = 1.27"
equation "\"Tool_Dia\" = 6.35"
body "Solid1"
